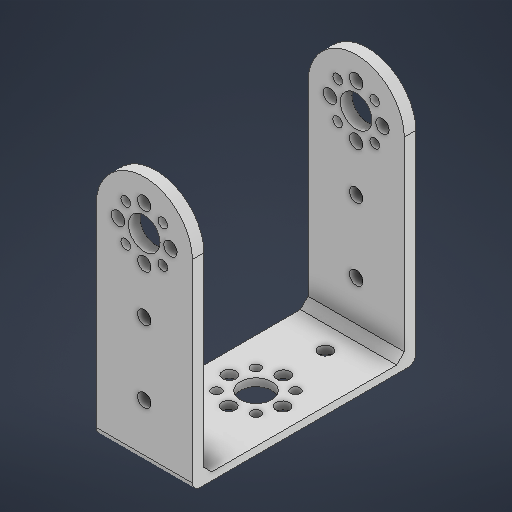
# Autodesk Inventor part: long FrameARRUMADO
Saved by Autodesk Inventor 2027 (Build 310192060, 192F)
## iProperties
Created: 2026-09-09
Part Number: long FrameARRUMADO
Material: Genérico
Document SubType Name: Modeling
Designer: joaop
Density: 1 g/cm^3
Appearance: Padrão
Author: joaop
Autodesk Inventor part; units mm, degrees
ref_plane "YZ Plane" through (0, 0, 0) normal (1, 0, 0) x (0, 1, 0)
ref_plane "XZ Plane" through (0, 0, 0) normal (0, 1, 0) x (-1, 0, 0)
ref_plane "XY Plane" through (0, 0, 0) normal (0, 0, 1) x (1, 0, 0)
sketch "Esboço1" plane through (0, 0, 0) normal (1, 0, 0) x (0, 1, 0)
  line L0 (0, 0) -> (64.55, 0)
  line L1 (64.55, 0) -> (64.55, 3)
  line L2 (64.55, 55) -> (64.55, 58)
  line L3 (64.55, 58) -> (0, 58)
  line L4 (0, 58) -> (0, 0)
  line L5 (0, 58) -> (0, 55)
  line L6 (2, 55) -> (2, 3)
  line L7 (2, 3) -> (64.55, 3)
  line L8 (2, 55) -> (64.55, 55)
  dimension "d6" = 64.55
  dimension "d7" = 58
  dimension "d81" = 64.55
  dimension "d83" = 2
  dimension "d84" = 52
  dimension "d85" = 62.55
  dimension "d86" = 62.55
  dimension "d111" = 3
  dimension "d112" = 3
  constraints: 18 end point, 3 perpendicular, 3 point on line, 1 horizontal
  measures "d6" distance of L2.end L3.end
  measures "d7" distance of L3.end L0.start
  measures "d81" distance of L0.start L0.end
  measures "d83" distance of L5.end L6.start
  measures "d84" distance of L6.start L6.end
  measures "d85" distance of L6.start L2.start
  measures "d86" distance of L6.end L1.end
  measures "d111" distance between parallel lines of L8 L3
  measures "d112" distance between parallel lines of L0 L7
extrude "Extrusão1" add sketch "Esboço1" along normal blind 25
sketch "Esboço2" plane through (0, 0, 58) normal (0, 0, 1) x (1, 0, 0)
  line L0 (0, 0) -> (25, 0)
  circle A0 centre (12.5, 14.4) radius 1.75
  circle A1 centre (12.5, 51.85) radius 4.1
  circle A2 centre (12.5, 45.05) radius 1.75
  line L1 (12.5, 51.85) -> (16.5, 51.85) construction
  line L2 (12.5, 51.85) -> (19.3, 51.85) construction
  circle A3 centre (7.691674, 47.041674) radius 1.25
  circle A4 centre (19.3, 51.85) radius 1.75
  circle A5 centre (12.5, 58.65) radius 1.75
  circle A6 centre (5.7, 51.85) radius 1.75
  circle A7 centre (17.308326, 47.041674) radius 1.25
  circle A8 centre (17.308326, 56.658326) radius 1.25
  circle A9 centre (7.691674, 56.658326) radius 1.25
  line L3 (0, 0) -> (25, 0)
  line L4 (25, 2) -> (25, 64.55)
  line L5 (0, 31) -> (0, 64.55)
  line L6 (0, 64.55) -> (25, 64.55)
  line L7 (25, 64.55) -> (25, 31)
  circle A10 centre (12.5, 33) radius 1.75
  line L8 (29.4167, 51.85) -> (-4.4167, 51.85)
  arc A11 (25, 51.85) -> (0, 51.85) centre (12.5, 52.048425) ccw
  point P0 (12.5, 0)
  point P1 (12.5, 64.55)
  point P2 (12.5, 0)
  point P3 (12.5, 0)
  point P4 (0, 52.24685)
  point P5 (25, 52.24685)
  dimension "d11" = 3.5
  dimension "d42" = 2.5
  dimension "d53" = 360
  dimension "d59" = 360
  dimension "d88" = 12.7
  dimension "d89" = 14.4
  dimension "d94" = 3.5
  dimension "d95" = 33
  dimension "d113" = 3.5
  dimension "d114" = 8.2
  constraints: 12 centre point, 12 end point, 5 midpoint, 5 point on line, 3 horizontal, 3 point on circle, 2 perpendicular, 1 vertical, 18 other
  measures "d11" diameter of A0
  measures "d42" diameter of A3
  measures "d88" distance from line of L6 L1.start
  measures "d89" distance of point (12.5, 0) A0.centre
  measures "d94" diameter of A10
  measures "d95" distance of point (12.5, 0) A10.centre
  measures "d113" diameter of A4
  measures "d114" diameter of A1
sketch "Esboço2 outline for Extrusão2" plane through (0, 0, 58) normal (0, 0, 1) x (1, 0, 0)
  circle A0 centre (12.5, 14.4) radius 1.75
  circle A1 centre (12.5, 51.85) radius 4.1
  circle A2 centre (12.5, 45.05) radius 1.75
  circle A3 centre (7.691674, 47.041674) radius 1.25
  circle A4 centre (17.308326, 47.041674) radius 1.25
  circle A5 centre (17.308326, 56.658326) radius 1.25
  circle A6 centre (12.5, 58.65) radius 1.75
  circle A7 centre (5.7, 51.85) radius 1.75
  circle A8 centre (7.691674, 56.658326) radius 1.25
  circle A9 centre (19.3, 51.85) radius 1.75
  circle A10 centre (12.5, 33) radius 1.75
  arc A11 (0, 52.24685) -> (12.5, 64.55) centre (12.5, 52.048425) cw
  line L0 (0, 64.55) -> (0, 52.24685)
  line L1 (12.5, 64.55) -> (0, 64.55)
  arc A12 (12.5, 64.55) -> (25, 52.24685) centre (12.5, 52.048425) cw
  line L2 (25, 64.55) -> (12.5, 64.55)
  line L3 (25, 52.24685) -> (25, 64.55)
extrude "Extrusão2" cut sketch "Esboço2 outline for Extrusão2" against normal through all
sketch "Esboço4" plane through (0, 0, 0) normal (0, -1, 0) x (1, 0, 0)
  line L0 (0, 58) -> (25, 58)
  line L1 (14.25, 0) -> (10.75, 0)
  line L2 (25, 2) -> (25, 54)
  line L3 (0, 2) -> (0, 54)
  circle A0 centre (12.5, 29) radius 4.1
  circle A1 centre (12.583333, 22) radius 1.75
  line L4 (12.5, 29) -> (16.5, 29) construction
  line L5 (12.5, 29) -> (19.3, 29) construction
  circle A2 centre (7.357232, 23.889772) radius 1.25
  circle A3 centre (19.5, 29.083333) radius 1.75
  circle A4 centre (12.416667, 36) radius 1.75
  circle A5 centre (5.5, 28.916667) radius 1.75
  circle A6 centre (17.610228, 23.857232) radius 1.25
  circle A7 centre (17.642768, 34.110228) radius 1.25
  circle A8 centre (7.389772, 34.142768) radius 1.25
  line L6 (0, 0) -> (25, 0)
  circle A9 centre (12.5, 47) radius 1.75
  circle A10 centre (12.5, 11) radius 1.75
  line L7 (25, 0) -> (25, 1)
  line L8 (25, 58) -> (25, 0)
  line L9 (25, 58) -> (25, 57)
  line L10 (25, 57) -> (25, 2)
  line L11 (12.5, 0) -> (12.5, 58)
  point P0 (24.956484, 28.030424)
  dimension "d68" = 8.2
  dimension "d69" = 3.5
  dimension "d70" = 2.5
  dimension "d72" = 360
  dimension "d74" = 360
  dimension "d97" = 29
  dimension "d109" = 3.5
  dimension "d110" = 3.5
  dimension "d118" = 11
  dimension "d124" = 11
  dimension "d125" = 5.5
  dimension "d126" = 5.5
  dimension "d127" = 12.5
  dimension "d128" = 12.5
  dimension "d129" = 12.5
  dimension "d130" = 12.5
  constraints: 12 end point, 11 centre point, 3 point on line, 2 horizontal, 2 midpoint, 1 collinear, 18 other
  measures "d68" diameter of A0
  measures "d69" diameter of A1
  measures "d70" diameter of A2
  measures "d97" distance from line of L0 L4.start
  measures "d109" diameter of A9
  measures "d110" diameter of A10
  measures "d118" vertical distance of A9.centre A4.centre
  measures "d124" vertical distance of A10.centre A1.centre
  measures "d125" distance from line of L3 A5.centre
  measures "d126" distance from line of L2 A3.centre
  measures "d127" distance between parallel lines of L3 L11
  measures "d128" distance from line of L8 point (12.5, 29)
  measures "d129" distance from line of L2 A10.centre
  measures "d130" distance from line of L2 A9.centre
extrude "Extrusão3" cut sketch "Esboço4" against normal through all contours L11 A9 | A9 L11 | L11 A4 | A4 L11 | L11 A0 | A0 L11 | L11 A1 | A1 L11 | L11 A10 | A10 L11 | A2 | A3 | A5 | A6 | A7 | A8
fillet "Arredondamento1" radius 2 2 edges at (12.5, 0, 0) (12.5, 0, 58)
chamfer "Chanfro1" distance 2 angle 45 2 edges at (12.5, 2, 55) (12.5, 2, 3)
